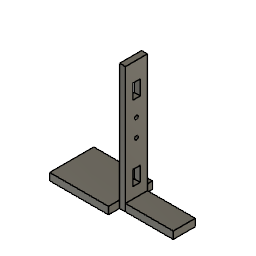
base (Autodesk Fusion 360 design; units mm, degrees)
Autodesk Fusion 360 part; units mm, degrees
sketch "Sketch1" plane through (0, 0, 0) normal (0, 1, 0) x (1, 0, 0)
  line L0 (-0.8925, -80) -> (7.1075, -80)
  line L1 (7.1075, -80) -> (7.1075, 91)
  line L2 (7.1075, 91) -> (-0.8925, 91)
  line L3 (-0.8925, 91) -> (-0.8925, -80)
  dimension "d1" = 8
  dimension "d2" = 171
  constraint horizontal L0
  constraint vertical L1
  constraint horizontal L2
  constraint vertical L3
  measures "d1" distance of L1 L3
  measures "d2" distance of L0.end L1.end
extrude "Extrude1" add sketch "Sketch1" along normal blind 30 makes body 1
sketch "Sketch2" plane through (0, 0, 0) normal (0, 1, 0) x (1, 0, 0)
  line L0 (291.3922, -10) -> (356.3922, -10)
  line L1 (356.3922, -10) -> (356.3922, 0)
  line L2 (356.3922, 0) -> (291.3922, 0)
  line L3 (291.3922, 0) -> (291.3922, -10)
  dimension "d5" = 10
  dimension "d6" = 65
  constraint horizontal L0
  constraint vertical L1
  constraint horizontal L2
  constraint vertical L3
  measures "d5" distance of L0 L2
  measures "d6" distance of L1.end L2.end
extrude "Extrude2" add sketch "Sketch2" along normal blind 30 separate body makes body 2
sketch "Sketch3" plane through (0, 0, 0) normal (0, 1, 0) x (1, 0, 0)
  line L0 (50, -10) -> (130, -10)
  line L1 (130, -10) -> (130, 0)
  line L2 (130, 0) -> (50, 0)
  line L3 (50, 0) -> (50, -10)
  dimension "d13" = 80
  dimension "d14" = 10
  constraint horizontal L0
  constraint vertical L1
  constraint horizontal L2
  constraint vertical L3
  measures "d13" distance of L1 L3
  measures "d14" distance of L0.end L1.end
extrude "Extrude3" add sketch "Sketch3" along normal blind 60 separate body makes body 3
copy_body "Body->Comp4" bodies 1 removing the originals makes body 4 in component "Component"
copy_body "Body->Comp5" bodies 2 removing the originals makes body 5 in component "base1"
copy_body "Body->Comp6" bodies 3 removing the originals makes body 6 in component "Component'"
sketch "Sketch6" plane through (291.3922, 0, -9) normal (1, 0, 0) x (0, 1, 0)
  line L0 (0, 180) -> (0, 9)
  line L1 (0, 9) -> (30, 9)
  line L2 (30, 9) -> (30, 180)
  line L3 (30, 180) -> (0, 180)
  line L4 (10.1844, 155.3906) -> (20.1844, 155.3906)
  line L5 (20.1844, 155.3906) -> (20.1844, 135.3906)
  line L6 (20.1844, 135.3906) -> (10.1844, 135.3906)
  line L7 (10.1844, 135.3906) -> (10.1844, 155.3906)
  line L8 (10.1134, 53.7758) -> (20.1134, 53.7758)
  line L9 (20.1134, 53.7758) -> (20.1134, 33.7758)
  line L10 (20.1134, 33.7758) -> (10.1134, 33.7758)
  line L11 (10.1134, 33.7758) -> (10.1134, 53.7758)
  dimension "d39" = 20
  dimension "d40" = 10
  dimension "d53" = 20
  dimension "d54" = 10
  constraint horizontal L4
  constraint vertical L5
  constraint horizontal L6
  constraint vertical L7
  constraint horizontal L8
  constraint vertical L9
  constraint horizontal L10
  constraint vertical L11
  measures "d39" distance of L8 L10
  measures "d40" distance of L9 L11
  measures "d53" distance of L4 L6
  measures "d54" distance of L5 L7
extrude "Extrude1'" cut sketch "Sketch6" against normal blind 10 contours L4 L5 L6 L7 | L8 L9 L10 L11 sketch seen with x (1, 0, 0) y (0, 1, 0) z (0, 0, 1) at (-284.2848, 0, -91) bodies 4 in component "Component"
sketch "Sketch7" plane through (283.3922, 0, 0) normal (-1, 0, 0) x (0, -1, 0)
  line L0 (-20.1844, 126.3906) -> (-20.1844, 146.3906)
  line L1 (-20.1844, 146.3906) -> (-10.1844, 146.3906)
  line L2 (-10.1844, 146.3906) -> (-10.1844, 126.3906)
  line L3 (-10.1844, 126.3906) -> (-20.1844, 126.3906)
  line L4 (-20.1134, 24.7758) -> (-20.1134, 44.7758)
  line L5 (-20.1134, 44.7758) -> (-10.1134, 44.7758)
  line L6 (-10.1134, 44.7758) -> (-10.1134, 24.7758)
  line L7 (-10.1134, 24.7758) -> (-20.1134, 24.7758)
  line L8 (0, 0) -> (0, 171)
  line L9 (0, 171) -> (-30, 171)
  line L10 (-30, 171) -> (-30, 0)
  line L11 (-30, 0) -> (0, 0)
  circle A0 centre (-15, 103.7757) radius 2.5
  circle A1 centre (-15, 79.7757) radius 2.5
  dimension "d59" = 5
  dimension "d60" = 5
  measures "d59" diameter of A0
  measures "d60" diameter of A1
extrude "Extrude2'" cut sketch "Sketch7" against normal blind 9 contours A0 | A1 sketch seen with x (1, 0, 0) y (0, 1, 0) z (0, 0, 1) at (-284.2848, 0, -91) bodies 4 in component "Component"
component "Component" placed x (1, 0, 0) y (0, 1, 0) z (0, 0, 1) at (284.2848, 0, 91)
component "base1" placed x (1, 0, 0) y (0, 1, 0) z (0, 0, 1) at (0, 0, 0)
component "Component'" placed x (1, 0, 0) y (0, 1, 0) z (0, 0, 1) at (153.3922, -15, 0)
named bodies: "base1"
